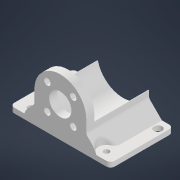
# Autodesk Inventor part: Gobilda 1620 motor mount
Saved by Autodesk Inventor 2022 (Build 260153000, 153)
## iProperties
Created: 2021-12-02
Part Number: Gobilda 1620 motor mount
Material: Generic
Document SubType Name: Modeling
Designer: izack
Density: 1 g/cm^3
Appearance: Default
Author: izack
Autodesk Inventor part; units mm, degrees
ref_plane "YZ Plane" through (0, 0, 0) normal (1, 0, 0) x (0, 1, 0)
ref_plane "XZ Plane" through (0, 0, 0) normal (0, 1, 0) x (-1, 0, 0)
ref_plane "XY Plane" through (0, 0, 0) normal (0, 0, 1) x (1, 0, 0)
sketch "Sketch1" plane through (0, 0, 0) normal (0, 0, 1) x (1, 0, 0)
  arc A0 (-6.4474, 9.2607) -> (-6.0115, 7.7857) centre (-8, 8) ccw
  arc A1 (-2.9419, 15.7272) -> (-15.7272, 2.9419) centre (0, 0) ccw
  arc A2 (2.9419, 15.7272) -> (-2.9419, 15.7272) centre (0, 0) ccw
  arc A3 (15.7272, 2.9419) -> (2.9419, 15.7272) centre (0, 0) ccw
  circle A4 centre (0, 0) radius 16
  circle A5 centre (-8, 8) radius 2
  arc A6 (9.2607, 6.4474) -> (7.7857, 6.0115) centre (8, 8) ccw
  arc A7 (6.4474, -9.2607) -> (6.0115, -7.7857) centre (8, -8) ccw
  arc A8 (-9.2607, -6.4474) -> (-7.7857, -6.0115) centre (-8, -8) ccw
  circle A9 centre (-8, -8) radius 2
  circle A10 centre (8, -8) radius 2
  circle A11 centre (8, 8) radius 2
  circle A12 centre (0, 0) radius 6.858
  line L0 (0, -16) -> (0, -19.0988)
  line L1 (0, -19.0988) -> (16, -19.0988)
  line L2 (16, -19.0988) -> (16, 0)
  line L3 (0, -19.0988) -> (-16, -19.0988)
  line L4 (-16, -19.0988) -> (-16, 0)
  line L5 (16, -19.0988) -> (31, -19.0988)
  line L6 (31, -19.0988) -> (31, -16)
  line L7 (31, -16) -> (16, -16)
  line L8 (16, -16) -> (16, -19.0988)
  line L9 (-16, -16) -> (-31, -16)
  line L10 (-31, -16) -> (-31, -19.0988)
  line L11 (-31, -19.0988) -> (-16, -19.0988)
  line L12 (-16, -19.0988) -> (-16, -16)
  point P0 (-15.7272, 2.9419)
  point P1 (-6.0115, 7.7857)
  point P2 (7.7857, 6.0115)
  point P3 (-7.7857, -6.0115)
extrude "Extrusion1" add sketch "Sketch1" along normal blind 5.0038
sketch "Sketch2" plane through (0, 0, 0) normal (0, 0, -1) x (-1, 0, 0)
  circle A0 centre (0, 0) radius 16
  line L0 (-16, -19.0988) -> (-16, 0) projected
  line L1 (-31, -16) -> (-16, -16) projected
  line L2 (-31, -19.0988) -> (-31, -16) projected
  line L3 (-16, -19.0988) -> (-31, -19.0988) projected
  line L4 (31, -19.0988) -> (-31, -19.0988) projected
  line L5 (31, -16) -> (31, -19.0988) projected
  line L6 (16, -16) -> (31, -16) projected
  line L7 (16, 0) -> (16, -16) projected
  constraints: 1 centre point, 1 coincident
ref_plane "Work Plane1" through (-15.805, -15.805, -33.75) normal (0, 0, 1) x (1, 0, 0)
extrude "Extrusion2" add sketch "Sketch2" along normal up to surface (33.75 mm away) contours L7 L6 L5 L4 L0 A0 | L0 L3 L2 L1
fillet "Fillet1" radius 0.254 2 edges at (16, 0, -16.875) (-16, 0, -16.875)
sketch "Sketch3" plane through (16, -16, 5.0038) normal (0, 1, 0) x (1, 0, 0)
  line L0 (-47, 0) -> (15, 0) construction
  line L1 (-32, 5.0038) -> (-32, 0) construction
  line L2 (-47, 0) -> (-32, 0) construction
  line L3 (-39.5, 0) -> (-39.5, 38.7538) construction
  line L4 (15, 38.7538) -> (-47, 38.7538) construction
  line L5 (0, 0) -> (15, 0) construction
  line L6 (7.5, 0) -> (7.5, 38.7538) construction
  line L7 (0, 38.7538) -> (15, 38.7538) construction
  circle A0 centre (-39.5, 5.0038) radius 1.7
  circle A1 centre (7.5, 5.0038) radius 1.7
  circle A2 centre (-39.5, 5.0038) radius 5
  circle A3 centre (7.5, 5.0038) radius 5
  point P0 (-16, 5.0038)
  dimension "d10" = 3.4
  dimension "d11" = 3.4
  dimension "d12" = 10
  dimension "d13" = 10
  constraints: 8 end point, 4 centre point, 3 midpoint, 3 point on line, 2 coincident, 1 horizontal, 1 perpendicular, 1 vertical
  measures "d10" diameter of A0
  measures "d11" diameter of A1
  measures "d12" diameter of A2
  measures "d13" diameter of A3
extrude "Extrusion3" cut sketch "Sketch3" against normal blind 25.4 contours A0 | A1
chamfer "Chamfer1" distance 7.9375 angle 45 2 edges at (-16, -16, -14.3731) (16, -16, -14.3731)
extrude "Extrusion4" cut sketch "Sketch3" along normal blind 25.4 contours A0 | A2 | A3
fillet "Fillet2" radius 2.54 3 edges at (18.5, -10.5625, 0) (-20.1227, -12.1852, -3.687) (-20.1227, -12.1852, 3.687)
fillet "Fillet3" radius 2.54 2 edges at (16, -8.0625, -14.3731) (-16, -8.0625, -14.3731)
fillet "Fillet4" radius 2.54 4 edges at (31, -17.5494, 5.0038) (31, -17.5494, -33.75) (-31, -17.5494, 5.0038) (-31, -17.5494, -33.75)
sketch "Sketch4" plane through (23.5, -16, 0) normal (0, 1, 0) x (1, 0, 0)
  line L0 (-54.5, 31.21) -> (-54.5, -2.4638) construction
  line L1 (-54.5, 28.1069) -> (7.5, 28.1069) construction
  line L2 (7.5, 31.21) -> (7.5, -2.4638) construction
  circle A0 centre (3.69, 28.1069) radius 2.5
  circle A1 centre (-50.69, 28.1069) radius 2.5
  point P0 (-23.5, 0)
  dimension "d24" = 5
  dimension "d25" = 5
  dimension "d26" = 3.81
  dimension "d27" = 3.81
  constraints: 4 point on line, 2 centre point, 2 end point, 1 horizontal
  measures "d24" diameter of A0
  measures "d25" diameter of A1
  measures "d26" distance from line of L2 A0.centre
  measures "d27" distance from line of L0 A1.centre
extrude "Extrusion5" cut sketch "Sketch4" against normal blind 25.4
body "Solid1"
